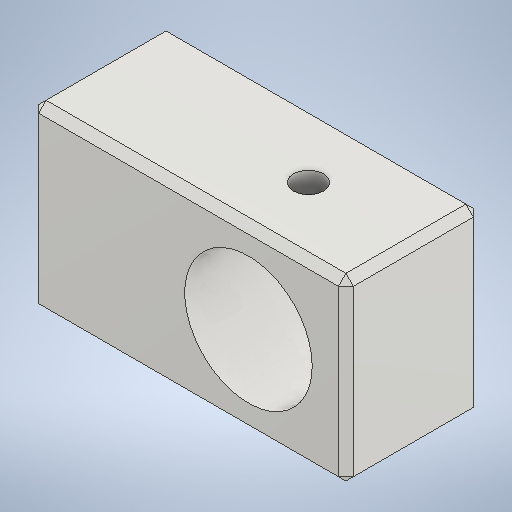
# Autodesk Inventor part: 16B2 - Con Head Big End
Saved by Autodesk Inventor 2025.2 (Build 292293000, 293)
## iProperties
Created: 2025-06-12
Part Number: 16B2 - Con Head Big End
Material: Steel AISI 1020 107 HR
Document SubType Name: Modeling
Designer: bless
Density: 7.87 g/cm^3
Appearance: Steel
Author: bless
Autodesk Inventor part; units mm, degrees
ref_plane "YZ Plane" through (0, 0, 0) normal (1, 0, 0) x (0, 1, 0)
ref_plane "XZ Plane" through (0, 0, 0) normal (0, 1, 0) x (-1, 0, 0)
ref_plane "XY Plane" through (0, 0, 0) normal (0, 0, 1) x (1, 0, 0)
sketch "Sketch1" plane through (0, 0, 0) normal (0, 0, 1) x (1, 0, 0)
  line L0 (-10.5, 6) -> (10.5, 6)
  line L1 (10.5, 6) -> (10.5, -6)
  line L2 (10.5, -6) -> (-10.5, -6)
  line L3 (-10.5, -6) -> (-10.5, 6)
  line L4 (-10.5, 6) -> (10.5, -6) construction
  line L5 (10.5, 6) -> (-10.5, -6) construction
  point P0 (0, 0)
  dimension "d0" = 21
  dimension "d1" = 12
  constraints: 12 end point, 2 midpoint, 2 parallel, 1 horizontal, 1 perpendicular
  measures "d0" distance of L0.start L0.end
  measures "d1" distance of L0.end L1.end
extrude "Extrusion1" add sketch "Sketch1" along normal blind 9
chamfer "Chamfer1" distance 0.5 angle 45 12 edges at (0, 6, 9) (-10.5, 0, 9) (10.5, 0, 9) (0, -6, 9) (10.5, 6, 4.5) (10.5, -6, 4.5) (10.5, 0, 0) (-10.5, 6, 4.5) (-10.5, -6, 4.5) (0, -6, 0) (-10.5, 0, 0) (0, 6, 0)
sketch "Sketch2" plane through (0, 0, 9) normal (0, 0, 1) x (1, 0, 0)
  circle A0 centre (4, 0) radius 4.25
  line L0 (10.5, -5.5) -> (10.5, 5.5) projected
  point P0 (0, 0)
  dimension "d7" = 8.5
  dimension "d8" = 6.5
  constraints: 1 centre point, 1 horizontal alignment
  measures "d7" diameter of A0
  measures "d8" distance from line of L0 A0.centre
extrude "Extrusion2" cut sketch "Sketch2" against normal through all
sketch "Sketch3" plane through (-10, 6, 0.5) normal (0, 1, 0) x (1, 0, 0)
  line L0 (20, 0) -> (20, -8) projected
  circle A0 centre (13.5, -4) radius 1
  point P0 (10, 0.5)
  point P1 (20, -4)
  point P2 (20, -4)
  dimension "d11" = 2
  dimension "d12" = 6.5
  constraints: 2 midpoint, 1 centre point, 1 horizontal alignment
  measures "d11" diameter of A0
  measures "d12" distance of point (20, -4) A0.centre
extrude "Extrusion3" cut sketch "Sketch3" against normal up to surface
sketch "Sketch4" plane through (-10.5, -5.5, 0.5) normal (-1, 0, 0) x (0, 0, 1)
  point P0 (-0.5, 5.5)
  point P1 (4, 5.5)
hole "Hole1" at (-10.5, 0, 4.5) direction (1, 0, 0) diameter 4.917 depth 10 thread size "M6x1" class "6H" standard "ANSI Metric M Profile"
body "Solid1"
